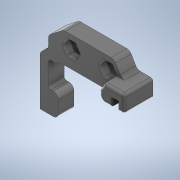
# Autodesk Inventor part: mount_battery
Saved by Autodesk Inventor 2022.2 (Build 262287000, 287)
## iProperties
Created: 2021-01-30
Part Number: mount_battery
Material: ABS Plastic
Document SubType Name: Modeling
Designer: User
Density: 1.06 g/cm^3
Appearance: Smooth - Black
Author: User
Autodesk Inventor part; units mm, degrees
ref_plane "YZ Plane" through (0, 0, 0) normal (1, 0, 0) x (0, 1, 0)
ref_plane "XZ Plane" through (0, 0, 0) normal (0, 1, 0) x (-1, 0, 0)
ref_plane "XY Plane" through (0, 0, 0) normal (0, 0, 1) x (1, 0, 0)
ref_plane "Work Plane1" through (0, 0, 0) normal (0, 0, 1) x (1, 0, 0)
sketch "mount_sketch" plane through (0, 0, 0) normal (0, 0, 1) x (1, 0, 0)
  circle A0 centre (42, 55.2584) radius 1.55 projected
  circle A1 centre (28, 55.2584) radius 1.55 projected
  line L0 (45, 60.2584) -> (25, 60.2584)
  line L1 (25, 60.2584) -> (15.4, 52.7584)
  line L2 (15.4, 52.7584) -> (15.4, 29.5584)
  line L3 (15.4, 29.5584) -> (19.4, 29.5584)
  line L4 (19.4, 29.5584) -> (19.4, 48.7584)
  line L5 (19.4, 48.7584) -> (23, 48.7584)
  circle A2 centre (42, -54.7416) radius 1.55 construction
  circle A3 centre (28, -54.7416) radius 1.55 construction
  line L6 (47, -54.627) -> (47, 66.2497) construction
  circle A4 centre (12, 51.2584) radius 1.55 construction
  circle A5 centre (12, -37.8416) radius 1.55 construction
  circle A6 centre (12, -54.7416) radius 1.55 construction
  circle A7 centre (29, -68.7416) radius 1.55 construction
  circle A8 centre (14, -68.7416) radius 1.55 construction
  line L7 (45, 50.2584) -> (25, 50.2584)
  line L8 (25, 50.2584) -> (23, 48.7584)
  line L9 (45, 60.2584) -> (46.5, 60.2584)
  line L10 (46.5, 60.2584) -> (46.5, 50.2584)
  line L11 (46.5, 50.2584) -> (45, 50.2584)
  line L12 (23, 48.7584) -> (23, 58.6959)
  line L13 (35, 55.2584) -> (35, 60.2584)
  line L14 (35, 55.2584) -> (35, 50.2584)
  line L15 (46.5, 60.2584) -> (50, 60.2584)
  line L16 (50, 60.2584) -> (50, 50.2584)
  line L17 (50, 50.2584) -> (46.5, 50.2584)
  line L18 (50, 60.2584) -> (56, 60.2584)
  line L19 (56, 60.2584) -> (56, 50.2584)
  line L20 (56, 50.2584) -> (50, 50.2584)
  line L21 (53, 50.2584) -> (56, 50.2584)
  line L22 (53, 50.2584) -> (53, 60.2584)
  point P0 (0, 0)
  dimension "d1" = 110
  dimension "d2" = 6.5
  dimension "d3" = 27.6
  dimension "d4" = 4
  dimension "d5" = 14
  dimension "d6" = 5
  dimension "d7" = 19.2
  dimension "d9" = 3.4
  dimension "d13" = 3
  dimension "d30" = 2
  dimension "d32" = 5
  dimension "d62" = 4.5
  dimension "d77" = 8
  dimension "d78" = 6
  constraints: 44 end point, 11 perpendicular, 4 horizontal, 4 midpoint, 2 vertical alignment, 1 collinear, 1 point on line, 1 vertical
  measures "d1" distance of A2.centre A0.centre
  measures "d2" distance from line of A0.centre L5
  measures "d3" distance between parallel lines of L6 L4
  measures "d4" distance between parallel lines of L4 L2
  measures "d5" vertical distance of A3.centre A7.centre
  measures "d6" distance from line of L0 A0.centre
  measures "d7" distance between parallel lines of L5 L3
  measures "d9" distance from line of L2 A4.centre
  measures "d13" horizontal distance of L0.end A1.centre
  measures "d30" horizontal distance of L0.end L5.end
  measures "d32" distance from line of L7 A0.centre
  measures "d62" distance from line of L10 A0.centre
  measures "d77" distance from line of L16 A0.centre
  measures "d78" distance of L19.end L16.end
extrude "mount" add sketch "mount_sketch" along normal blind 6 contours L9 L10 L11 L7 L14 L13 L0 | L13 L14 L7 L8 L12 L1 L0 | L12 L5 L4 L3 L2 L1
fillet "common" radius 2 2 edges at (25, 60.2584, 3) (25, 50.2584, 3)
sketch "nuts_sketch" plane through (0, 0, 6) normal (0, 0, 1) x (1, 0, 0)
  circle A0 centre (42, 55.2584) radius 1.55 projected
  circle A1 centre (28, 55.2584) radius 1.55 projected
  line L0 (38.4782, 55.2584) -> (40.2391, 58.3084)
  line L1 (40.2391, 58.3084) -> (43.7609, 58.3084)
  line L2 (43.7609, 58.3084) -> (45.5218, 55.2584)
  line L3 (45.5218, 55.2584) -> (43.7609, 52.2084)
  line L4 (43.7609, 52.2084) -> (40.2391, 52.2084)
  line L5 (40.2391, 52.2084) -> (38.4782, 55.2584)
  line L6 (31.5218, 55.2584) -> (29.7609, 52.2084)
  line L7 (29.7609, 52.2084) -> (26.2391, 52.2084)
  line L8 (26.2391, 52.2084) -> (24.4782, 55.2584)
  line L9 (24.4782, 55.2584) -> (26.2391, 58.3084)
  line L10 (26.2391, 58.3084) -> (29.7609, 58.3084)
  line L11 (29.7609, 58.3084) -> (31.5218, 55.2584)
  point P0 (0, 0)
  dimension "d26" = 6.1
  dimension "d27" = 6.1
  constraints: 24 end point, 2 coincident, 2 horizontal alignment, 26 other
  measures "d26" distance between parallel lines of L2 L5
  measures "d27" distance between parallel lines of L8 L11
extrude "nuts" cut sketch "nuts_sketch" against normal blind 3
sketch "Sketch13" plane through (46.5, 50.2584, 0) normal (1, 0, 0) x (0, 0, -1)
  line L0 (0, 10) -> (-6, 10) projected
  line L1 (0, 0) -> (-6, 0) projected
  line L2 (-6, 10) -> (-6, 0)
  line L3 (0, 0) -> (0, 10) projected
  line L4 (-6, 0) -> (0, 0)
  line L5 (0, 0) -> (0, 10)
  line L6 (0, 10) -> (-6, 10)
  point P0 (0, -50.2584)
  constraints: 8 end point, 3 perpendicular, 1 vertical
extrude "Extrusion11" add sketch "Sketch13" along normal blind 9.5
sketch "Sketch20" plane through (19.4, 29.5584, 0) normal (1, 0, 0) x (0, 0, -1)
  line L0 (-6, 0) -> (-6, 19.2) projected
  line L1 (-6, 0) -> (-6, 19.2)
  line L2 (0, 19.2) -> (-6, 19.2) projected
  line L3 (-6, 19.2) -> (0, 19.2)
  line L4 (0, 0) -> (-6, 0) projected
  line L5 (0, 19.2) -> (0, 0)
  line L6 (0, 0) -> (-6, 0)
  point P0 (0, -29.5584)
  constraints: 8 end point, 2 collinear, 1 perpendicular, 1 vertical
extrude "Extrusion15" add sketch "Sketch20" along normal blind 3.6
sketch "Sketch21" plane through (0, 0, 6) normal (0, 0, 1) x (1, 0, 0)
  line L0 (15.4, 29.5584) -> (23, 29.5584) projected
  line L1 (19.2, 29.5584) -> (19.2, 55.7272)
  line L2 (24.4573, 59.8345) -> (15.4, 52.7584) projected
  line L3 (15.4, 52.7584) -> (15.4, 29.5584) projected
  line L4 (19.2, 29.5584) -> (15.4, 29.5584)
  line L5 (15.4, 29.5584) -> (15.4, 52.7584)
  line L6 (15.4, 52.7584) -> (19.2, 55.7272)
  line L7 (23, 48.7584) -> (24.4667, 49.8584) projected
  line L8 (23, 48.7584) -> (19.2, 48.7584)
  line L9 (23, 48.7584) -> (23, 29.5584) projected
  line L10 (23, 48.7584) -> (23, 58.6959)
  line L11 (19.2, 48.7584) -> (23, 58.6959)
  point P0 (0, 0)
  constraints: 14 end point, 3 point on line, 2 vertical, 1 collinear, 1 horizontal, 1 midpoint, 1 perpendicular
extrude "Extrusion16" cut sketch "Sketch21" against normal blind 6 contours L3 L2 L1 L0
fillet "Fillet13" radius 2 1 edges at (23, 48.7584, 3)
sketch "Sketch27" plane through (25.6667, 50.2584, 0) normal (0, -1, 0) x (1, 0, 0)
  line L0 (0, 0) -> (0, 6) projected
  line L1 (0, 0) -> (30.3333, 0) projected
  line L2 (30.3333, 6) -> (30.3333, 0) projected
  line L3 (0, 6) -> (30.3333, 6) projected
  point P0 (-25.6667, 0)
extrude "Extrusion21" add sketch "Sketch27" along normal blind 1.5
sketch "Sketch28" plane through (25.6667, 48.7584, 0) normal (-1, 0, 0) x (0, 0, 1)
  line L0 (0, 1.5) -> (6, 1.5) projected
  line L1 (0, 1.5) -> (0, 0) projected
  line L2 (6, 0) -> (0, 0) projected
  line L3 (6, 1.5) -> (6, 0) projected
  point P0 (0, -48.7584)
extrude "Extrusion22" add sketch "Sketch28" along normal through all
sketch "Sketch29" plane through (0, 0, 6) normal (0, 0, 1) x (1, 0, 0)
  line L0 (24.4782, 55.2584) -> (26.2391, 58.3084) projected
  line L1 (26.2391, 58.3084) -> (29.7609, 58.3084) projected
  line L2 (29.7609, 58.3084) -> (31.5218, 55.2584) projected
  line L3 (31.5218, 55.2584) -> (29.7609, 52.2084) projected
  line L4 (29.7609, 52.2084) -> (26.2391, 52.2084) projected
  line L5 (26.2391, 52.2084) -> (24.4782, 55.2584) projected
  line L6 (45.5218, 55.2584) -> (43.7609, 52.2084) projected
  line L7 (43.7609, 52.2084) -> (40.2391, 52.2084) projected
  line L8 (40.2391, 52.2084) -> (38.4782, 55.2584) projected
  line L9 (38.4782, 55.2584) -> (40.2391, 58.3084) projected
  line L10 (40.2391, 58.3084) -> (43.7609, 58.3084) projected
  line L11 (43.7609, 58.3084) -> (45.5218, 55.2584) projected
  line L12 (19.2, 55.7272) -> (19.2, 29.5584) projected
  line L13 (23, 47.7584) -> (23, 29.5584) projected
  line L14 (56, 48.7584) -> (23.2679, 48.7584) projected
  line L15 (56, 60.2584) -> (56, 48.7584) projected
  line L16 (25.6886, 60.2584) -> (56, 60.2584) projected
  arc A0 (25.6886, 60.2584) -> (24.4573, 59.8345) centre (25.6886, 58.2584) ccw projected
  line L17 (24.4573, 59.8345) -> (19.2, 55.7272) projected
  line L18 (45.5218, 55.2584) -> (56, 55.2584)
  line L19 (56, 60.2584) -> (56, 48.7584) projected
  line L20 (43.7609, 58.3084) -> (45.5218, 55.2584) projected
  line L21 (45.5218, 55.2584) -> (45.5218, 48.7584)
  line L22 (45.5218, 55.2584) -> (45.5218, 60.2584)
  line L23 (43.7609, 58.3084) -> (43.7609, 60.2584)
  line L24 (43.7609, 52.2084) -> (43.7609, 48.7584)
  line L25 (43.7609, 60.2584) -> (45.5218, 60.2584)
  line L26 (25.6886, 60.2584) -> (56, 60.2584) projected
  line L27 (45.5218, 60.2584) -> (47.2828, 60.2584)
  line L28 (47.2828, 60.2584) -> (47.2828, 48.7584)
  line L29 (45.5218, 55.2584) -> (43.7609, 52.2084) projected
  line L30 (43.7609, 52.2084) -> (56, 52.2084)
  line L31 (56, 60.2584) -> (56, 48.7584) projected
  line L32 (47.2828, 55.2584) -> (44.396, 60.2584)
  line L33 (47.2828, 48.7584) -> (53.2828, 48.7584)
  line L34 (53.2828, 48.7584) -> (53.2828, 60.2584)
  line L35 (53.2828, 60.2584) -> (47.2828, 60.2584)
  line L36 (47.2828, 60.2584) -> (47.2828, 48.7584)
  arc A1 (23.2679, 48.7584) -> (23, 47.7584) centre (25, 47.7584) ccw projected
  line L37 (19.2, 29.5584) -> (23, 29.5584) projected
  point P0 (0, 0)
  point P1 (53.2828, 55.2584)
  dimension "d139" = 6
  dimension "d140" = 11.5
  constraints: 28 end point, 12 point on line, 6 perpendicular, 3 parallel, 2 collinear, 2 horizontal
  measures "d139" distance of L34.end L35.end
  measures "d140" distance of L33.end L34.end
extrude "Extrusion24" add sketch "Sketch29" along normal blind 5 contours L21 L30 L6 | L18 L28 L30 L21 | L30 L21 L14 L24 | L18 L34 L30 L28 | L30 L28 L14 L21 | L30 L34 L14 L28
sketch "Sketch30" plane through (25.6667, 48.7584, 0) normal (0, -1, 0) x (1, 0, 0)
  line L0 (30.3333, 0) -> (-2.3987, 0) projected
  line L1 (30.3333, 0) -> (30.3333, 6) projected
  line L2 (18.0943, 6) -> (-2.3987, 6) projected
  line L3 (18.0943, 11) -> (27.6161, 11) projected
  line L4 (22.6943, 11) -> (25.3943, 11)
  line L5 (25.3943, 11) -> (25.3943, 3)
  line L6 (25.3943, 3) -> (22.6943, 3)
  line L7 (22.6943, 3) -> (22.6943, 11)
  line L8 (18.0943, 11) -> (27.6161, 11) projected
  line L9 (18.0943, 6) -> (18.0943, 11) projected
  line L10 (30.3333, 6) -> (27.6161, 6) projected
  line L11 (27.6161, 6) -> (27.6161, 11) projected
  line L12 (-2.3987, 0) -> (-2.3987, 6) projected
  point P0 (-25.6667, 0)
  point P1 (30.3333, 11)
  dimension "d132" = 2.7
  dimension "d134" = 4.6
  constraints: 8 end point, 2 parallel, 1 horizontal, 1 perpendicular, 1 point on line
  measures "d132" distance of L5.end L6.end
  measures "d134" distance between parallel lines of L9 L7
extrude "Extrusion25" cut sketch "Sketch30" against normal blind 3.45 contours L5 L6 L7 L3
fillet "Fillet20" radius 1 1 edges at (49.7109, 52.2084, 3)
extrude "Extrusion26" cut sketch "Sketch29" against normal through all contours L28 L16 L34 L18 | L32 L22 L16 L28 | L32 L16 L22 | L34 L16 L15 L18
fillet "Fillet21" radius 2 3 edges at (44.396, 60.2584, 3) (47.2828, 55.2584, 3) (43.7609, 48.7584, 8.5)
fillet "Fillet22" radius 1 6 edges at (52.1718, 48.7584, 11) (47.0609, 48.7584, 11) (49.4023, 55.2584, 11) (43.7609, 51.4834, 11) (44.3467, 49.3442, 11) (44.6414, 53.7334, 11)
extrude "Extrusion27" cut sketch "Sketch29" against normal through all contours L18 L15 L30 L34 | L30 L15 L14 L34
fillet "Fillet23" radius 1 5 edges at (53.2828, 54.9655, 10.7071) (53.2828, 52.0084, 11) (53.2828, 49.0513, 10.7071) (53.2828, 48.7584, 5) (53.2828, 55.2584, 5)
sketch "Sketch32" plane through (0, 0, 6) normal (0, 0, 1) x (1, 0, 0)
  arc A0 (44.9734, 59.2584) -> (43.2413, 60.2584) centre (43.2413, 58.2584) ccw projected
  line L0 (25.6886, 60.2584) -> (43.2413, 60.2584) projected
  arc A1 (25.6886, 60.2584) -> (24.4573, 59.8345) centre (25.6886, 58.2584) ccw projected
  line L1 (24.4573, 59.8345) -> (19.2, 55.7272) projected
  line L2 (19.2, 55.7272) -> (19.2, 29.5584) projected
  line L3 (23, 47.7584) -> (23, 29.5584) projected
  line L4 (45.7609, 48.7584) -> (23.2679, 48.7584) projected
  arc A2 (43.7609, 50.7584) -> (45.7609, 48.7584) centre (45.7609, 50.7584) ccw projected
  line L5 (43.7609, 50.7584) -> (43.7609, 52.2084) projected
  line L6 (43.7609, 52.2084) -> (40.2391, 52.2084) projected
  line L7 (40.2391, 52.2084) -> (38.4782, 55.2584) projected
  line L8 (38.4782, 55.2584) -> (40.2391, 58.3084) projected
  line L9 (40.2391, 58.3084) -> (43.7609, 58.3084) projected
  line L10 (43.7609, 58.3084) -> (45.5218, 55.2584) projected
  line L11 (45.5218, 55.2584) -> (48.4375, 55.2584) projected
  arc A3 (46.7054, 56.2584) -> (48.4375, 55.2584) centre (48.4375, 57.2584) ccw projected
  line L12 (46.7054, 56.2584) -> (44.9734, 59.2584) projected
  line L13 (24.4782, 55.2584) -> (26.2391, 58.3084) projected
  line L14 (26.2391, 58.3084) -> (29.7609, 58.3084) projected
  line L15 (29.7609, 58.3084) -> (31.5218, 55.2584) projected
  line L16 (31.5218, 55.2584) -> (29.7609, 52.2084) projected
  line L17 (29.7609, 52.2084) -> (26.2391, 52.2084) projected
  line L18 (26.2391, 52.2084) -> (24.4782, 55.2584) projected
  line L19 (23, 47.7584) -> (23, 31.5584) projected
  line L20 (19.2, 54.7517) -> (19.2, 31.5484) projected
  line L21 (23, 31.5584) -> (19.2, 31.5584)
  line L22 (19.2, 31.5584) -> (19.2, 47.7584)
  line L23 (19.2, 47.7584) -> (23, 47.7584)
  line L24 (23, 47.7584) -> (23, 31.5584)
  arc A4 (19.9687, 56.3277) -> (19.2, 54.7517) centre (21.2, 54.7517) ccw projected
  line L25 (23, 47.7584) -> (19.2, 47.7584)
  line L26 (19.2, 47.7584) -> (19.2, 54.7517)
  line L27 (19.2, 54.7517) -> (23, 54.7517)
  line L28 (23, 54.7517) -> (23, 47.7584)
  line L29 (19.2, 54.7517) -> (16, 54.7517)
  line L30 (16, 54.7517) -> (16, 35.4604)
  line L31 (16, 35.4604) -> (19.2, 35.4604)
  line L32 (19.2, 35.4604) -> (19.2, 54.7517)
  line L33 (19.2, 31.5848) -> (19.2, 38.0185)
  line L34 (19.2, 38.0185) -> (23, 38.0185)
  arc A5 (23.2679, 48.7584) -> (23, 47.7584) centre (25, 47.7584) ccw projected
  line L35 (19.2, 29.5584) -> (23, 29.5584) projected
  line L36 (19.2, 54.7517) -> (16, 54.7517)
  line L37 (16, 54.7517) -> (16, 52.2084)
  line L38 (16, 52.2084) -> (19.2, 52.2084)
  line L39 (19.2, 52.2084) -> (19.2, 54.7517)
  line L40 (19.2, 54.7517) -> (16, 54.7517)
  line L41 (16, 54.7517) -> (16, 50.3636)
  line L42 (16, 50.3636) -> (19.2, 50.3636)
  line L43 (19.2, 50.3636) -> (19.2, 54.7517)
  point P0 (0, 0)
  dimension "d146" = 6.4337
  constraints: 44 end point, 10 parallel, 6 perpendicular, 5 horizontal, 5 point on line, 1 collinear
  measures "d146" distance of L33.start L33.end
extrude "Extrusion28" add sketch "Sketch32" against normal blind 6 contours L2 L38 L30 L29 | L2 L42 L30 L38 | L2 L31 L30 L42
extrude "Extrusion29" cut sketch "Sketch32" against normal through all contours L2 L38 L30 L29 | L2 L42 L30 L38 | L3 L34 L2 L23
sketch "Sketch33" plane through (16, 35.4604, 6) normal (0, -1, 0) x (1, 0, 0)
  line L0 (0, 0) -> (3.2, 0) projected
  line L1 (0, 0) -> (0, -6) projected
  line L2 (3.2, -6) -> (0, -6) projected
  line L3 (3.2, 0) -> (3.2, -6) projected
  point P0 (-16, -6)
extrude "Extrusion30" add sketch "Sketch33" along normal up to surface (5.902 mm away)
fillet "Fillet24" radius 2 4 edges at (23, 29.5584, 3) (23, 38.0185, 3) (23, 47.7584, 3) (19.2, 55.7272, 3)
fillet "Fillet25" radius 1 2 edges at (19.2, 47.7584, 3) (19.2, 38.0185, 3)
chamfer "Chamfer1" distance 2 angle 45 1 edges at (16, 50.3636, 3)
fillet "Fillet26" radius 2 3 edges at (19.2, 50.3636, 3) (16, 48.3636, 3) (18, 50.3636, 3)
chamfer "Chamfer2" distance 1 distance2 0.1 3 edges at (51.0609, 48.7584, 6.5) (51.0609, 49.0513, 10.7071) (51.0609, 50.9834, 11) measured on face at (51.0609, 49.4049, 10.3536) measured on face at (51.0609, 49.2584, 6.5) measured on face at (51.0609, 50.9834, 10.5)
chamfer "Chamfer3" distance 1 distance2 0.1 3 edges at (48.3609, 48.7584, 6.5) (48.3609, 49.0513, 10.7071) (48.3609, 50.9834, 11) measured on face at (48.3609, 49.2584, 6.5) measured on face at (48.3609, 49.4049, 10.3536) measured on face at (48.3609, 50.9834, 10.5)
equation "\"d27\" = d26"
body "Solid1"
